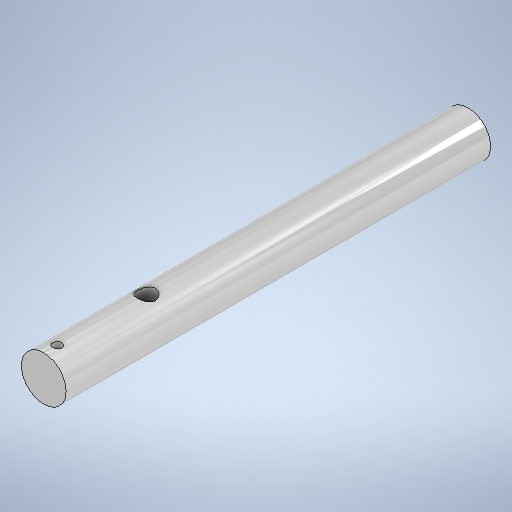
# Autodesk Inventor part: light_bar_roller_10
Saved by Autodesk Inventor 2025.1 (Build 291241000, 241)
## iProperties
Created: 2022-02-06
Part Number: light_bar_roller_10
Material: アルミニウム 6061-AHC
Document SubType Name: Modeling
Designer: 中島 青蔵
Density: 2.7 g/cm^3
Appearance: アルミニウム - ダーク
Author: 中島 青蔵
Autodesk Inventor part; units mm, degrees
ref_plane "YZ Plane" through (0, 0, 0) normal (1, 0, 0) x (0, 1, 0)
ref_plane "XY Plane" through (0, 0, 0) normal (0, 0, 1) x (1, 0, 0)
sketch "スケッチ1" plane through (0, 0, 0) normal (0, 0, 1) x (1, 0, 0)
  circle A0 centre (0, 0) radius 5
  dimension "d0" = 10
  constraints: 1 centre point, 1 coincident
  measures "d0" diameter of A0
extrude "押し出し1" add sketch "スケッチ1" along normal blind 137
ref_plane "作業平面1" through (0, 5, 0) normal (0, 1, 0) x (-1, 0, 0)
sketch "スケッチ2" plane through (0, 5, 0) normal (0, 1, 0) x (-1, 0, 0)
  line L0 (5, 0) -> (-5, 0) projected
  line L1 (5, 137) -> (-5, 137) projected
  point P0 (0, 0)
  point P1 (0, 3)
  point P2 (0, 134)
  point P3 (0, 114)
  point P4 (0, 38)
  point P5 (0, 69.5)
  point P6 (0, 50)
  dimension "d3" = 3
  dimension "d19" = 3
  dimension "d20" = 23
  dimension "d22" = 99
  dimension "d23" = 44.5
  dimension "d24" = 19.5
  measures "d3" distance from line of L0 point (0, 3)
  measures "d19" distance from line of L1 point (0, 134)
  measures "d20" distance from line of L1 point (0, 114)
  measures "d22" distance from line of L1 point (0, 38)
  measures "d23" distance of point (0, 114) point (0, 69.5)
  measures "d24" distance of point (0, 69.5) point (0, 50)
hole "穴1" at (0, 5, 3) at (0, 5, 134) at (0, 5, 38) direction (0, -1, 0) diameter 2 end through all
hole "穴2" at (0, 5, 114) direction (0, -1, 0) diameter 4 end through all
sketch "スケッチ4" plane through (0, 0, 0) normal (0, 0, -1) x (-1, 0, 0)
  circle A0 centre (0, 0) radius 5 projected
  circle A1 centre (0, 0) radius 5
  constraints: 1 centre point, 1 coincident, 1 concentric
extrude "押し出し2" cut sketch "スケッチ4" against normal blind 42
